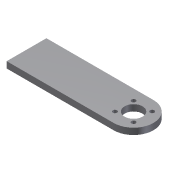
# Autodesk Inventor part: JointC4
Saved by Autodesk Inventor 2011 SP1 (Build 150282100, 282)
## iProperties
Created: 2012-10-23
Part Number: JointC4
Document SubType Name: Modeling
Designer: arihon
Density: 1 g/cm^3
Author: arihon
Autodesk Inventor part; units mm, degrees
ref_plane "YZ Plane" through (0, 0, 0) normal (1, 0, 0) x (0, 1, 0)
ref_plane "XZ Plane" through (0, 0, 0) normal (0, 1, 0) x (-1, 0, 0)
ref_plane "XY Plane" through (0, 0, 0) normal (0, 0, 1) x (1, 0, 0)
sketch "スケッチ1" plane through (0, 0, 0) normal (0, 0, 1) x (1, 0, 0)
  line L0 (-30, 9.4) -> (30, 9.4)
  line L1 (30, 9.4) -> (30, -9.4)
  line L2 (30, -9.4) -> (-30, -9.4)
  line L3 (-30, -9.4) -> (-30, 9.4)
  line L4 (30, 0) -> (-30, 0)
  circle A0 centre (16.2, 4.4) radius 1
  circle A1 centre (25, 4.4) radius 1
  circle A2 centre (16.2, -4.4) radius 1
  circle A3 centre (25, -4.4) radius 1
  point P0 (0, 0)
  dimension "d0" = 60
  dimension "d1" = 18.8
  dimension "d2" = 9.4
  dimension "d3" = 30
  dimension "d4" = 8.8
  dimension "d5" = 8.8
  dimension "d6" = 8.8
  dimension "d7" = 8.8
  dimension "d8" = 8.8
  dimension "d9" = 5
  dimension "d10" = 2
  dimension "d11" = 2
  dimension "d12" = 2
  dimension "d13" = 2
  constraints: 10 end point, 4 centre point, 4 coincident, 2 midpoint, 2 parallel, 1 horizontal, 1 perpendicular
  measures "d0" distance of L1.end L2.end
  measures "d1" distance of L2.end L0.start
  measures "d2" distance from line of L2 point (0, 0)
  measures "d3" distance from line of L3 point (0, 0)
  measures "d4" distance of point (16.2, 4.4) point (25, 4.4)
  measures "d5" distance of point (16.2, -4.4) point (25, -4.4)
  measures "d6" distance of point (25, -4.4) point (25, 4.4)
  measures "d7" distance of point (16.2, -4.4) point (16.2, 4.4)
  measures "d8" diameter of point (25, -4.4) L4
  measures "d9" distance from line of L1 point (25, -4.4)
  measures "d10" diameter of A0
  measures "d11" diameter of A1
  measures "d12" diameter of A2
  measures "d13" diameter of A3
extrude "押し出し1" add sketch "スケッチ1" along normal blind 3
fillet "フィレット1" radius 9.4 2 edges at (30, 9.4, 1.5) (30, -9.4, 1.5)
sketch "スケッチ2" plane through (0, 0, 3) normal (0, 0, 1) x (1, 0, 0)
  arc A0 (20.6, -9.4) -> (20.6, 9.4) centre (20.6, 0) ccw projected
  circle A1 centre (20.6, 0) radius 4.25
  point P0 (0, 0)
  dimension "d17" = 8.5
  constraints: 1 centre point, 1 coincident
  measures "d17" diameter of A1
extrude "押し出し2" cut sketch "スケッチ2" against normal through all
equation "\"d2\" = 0.5 * d1"
equation "\"d3\" = 0.5 * d0"
equation "\"d5\" = d4"
equation "\"d6\" = d4"
equation "\"d7\" = d4"
equation "\"d8\" = d4"
